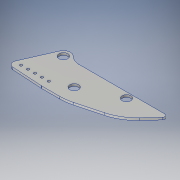
# Autodesk Inventor part: Flywheel Bracket 1
Saved by Autodesk Inventor 2019.4 (Build 234330000, 330)
## iProperties
Created: 2020-01-06
Part Number: Flywheel Bracket 1
Material: Aluminum 6061
Document SubType Name: Modeling
Designer: admin
Density: 2.7 g/cm^3
Appearance: Aluminum - Flat
Author: admin
Autodesk Inventor part; units mm, degrees
ref_plane "YZ Plane" through (0, 0, 0) normal (1, 0, 0) x (0, 1, 0)
ref_plane "XZ Plane" through (0, 0, 0) normal (0, 1, 0) x (-1, 0, 0)
ref_plane "XY Plane" through (0, 0, 0) normal (0, 0, 1) x (1, 0, 0)
sketch "Sketch1" plane through (0, 0, 0) normal (0, 1, 0) x (-1, 0, 0)
  circle A0 centre (0, 0) radius 9.5
  circle A1 centre (77.0362, 35.9226) radius 9.5
  line L0 (77.0362, 35.9226) -> (0, 0) construction
  line L1 (114.6028, -12) -> (-82.3554, -12)
  line L2 (-82.3554, -12) -> (-31.0868, 43.4655)
  line L3 (-31.0868, 43.4655) -> (62.6574, 68.4226)
  line L4 (62.6574, 68.4226) -> (115.432, 68.4226)
  arc A2 (109.5362, 35.9226) -> (85.4876, 4.5407) centre (77.0362, 35.9226) ccw construction
  circle A3 centre (0, 0) radius 40
  circle A4 centre (146.6896, -10.4495) radius 9.5
  circle A5 centre (146.6896, -10.4495) radius 15
  arc A6 (135.994, -20.9663) -> (114.6028, -12) centre (114.6028, -42) ccw
  line L5 (160.432, -16.4618) -> (195.432, 63.5382)
  line L6 (195.432, 63.5382) -> (115.432, 68.4226)
  dimension "d0" = 19
  dimension "d1" = 19
  dimension "d2" = 85
  dimension "d3" = 65
  dimension "d4" = 80
  dimension "d5" = 12
  dimension "d6" = 50
  dimension "d7" = 25
  dimension "d12" = 19
  dimension "d13" = 30
  dimension "d14" = 30
  dimension "d16" = 35
  dimension "d17" = 80
  dimension "d18" = 80
  constraints: 14 end point, 7 centre point, 6 point on circle, 5 coincident, 4 tangent, 1 horizontal, 1 parallel, 1 other
  measures "d0" diameter of A0
  measures "d1" diameter of A1
  measures "d2" distance of L0.start L0.end
  measures "d3" diameter of A2
  measures "d4" diameter of A3
  measures "d5" distance from line of L0.end L1
  measures "d6" distance from line of A3.centre L3
  measures "d7" angle of L1 L0
  measures "d12" diameter of A4
  measures "d13" diameter of A5
  measures "d14" radius of A6
  measures "d16" horizontal distance of L5.start L5.end
  measures "d17" vertical distance of L5.start L5.end
  measures "d18" horizontal distance of L5.end L4.end
extrude "Extrusion1" add sketch "Sketch1" along normal blind 5 contours L1 A3 L2 L3 L4 L6 L5 A5 A6 | L1 A3 | A5 picked at (-13.2582, 26.5327)
fillet "Fillet1" radius 5 1 edges at (82.3554, 2.5, -12)
fillet "Fillet2" radius 100 3 edges at (31.0868, 2.5, 43.4655) (-62.6574, 2.5, 68.4226) (-114.6028, 2.5, -12)
fillet "Fillet3" radius 10 2 edges at (-195.432, 2.5, 63.5382) (-115.432, 2.5, 68.4226)
sketch "Sketch2" plane through (0, 5, 0) normal (0, 1, 0) x (1, 0, 0)
  circle A0 centre (-160.5317, -51.9293) radius 2.75
  circle A1 centre (-145.5317, -51.9293) radius 2.75
  circle A2 centre (-130.5317, -51.9293) radius 2.75
  circle A3 centre (-115.5317, -51.9293) radius 2.75
  arc A4 (-189.6932, -50.4212) -> (-181.1411, -64.4108) centre (-180.5317, -54.4293) ccw projected
  circle A5 centre (-175.5317, -51.9293) radius 2.75
  point P0 (0, 0)
  dimension "d19" = 5.5
  dimension "d20" = 5.5
  dimension "d21" = 5.5
  dimension "d22" = 5.5
  dimension "d23" = 15
  dimension "d24" = 15
  dimension "d25" = 15
  dimension "d26" = 20
  dimension "d27" = 2.5
  dimension "d28" = 2.5
  dimension "d29" = 2.5
  dimension "d30" = 2.5
  dimension "d33" = 5.5
  dimension "d34" = 15
  dimension "d35" = 2.5
  constraints: 5 centre point
  measures "d19" diameter of A0
  measures "d20" diameter of A1
  measures "d21" diameter of A2
  measures "d22" diameter of A3
  measures "d23" distance of A2.centre A3.centre
  measures "d24" distance of A1.centre A2.centre
  measures "d25" distance of A1.centre A0.centre
  measures "d26" horizontal distance of A0.centre A4.centre
  measures "d27" vertical distance of A4.centre A0.centre
  measures "d28" vertical distance of A4.centre A1.centre
  measures "d29" vertical distance of A4.centre A2.centre
  measures "d30" vertical distance of A4.centre A3.centre
  measures "d33" diameter of A5
  measures "d34" distance of A0.centre A5.centre
  measures "d35" vertical distance of A4.centre A5.centre
extrude "Extrusion2" cut sketch "Sketch2" against normal through all
body "Solid1"
